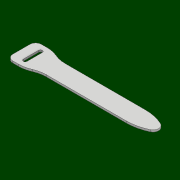
# Autodesk Inventor part: fastener_strap_t1
Saved by Autodesk Inventor 2018 (Build 220112000, 112)
## iProperties
Created: 2021-12-05
Part Number: fastener_strap_t1
Material: 一般
Document SubType Name: Modeling
Designer: gisen
Density: 1 g/cm^3
Appearance: 既定
Author: gisen
Autodesk Inventor part; units mm, degrees
ref_plane "YZ Plane" through (0, 0, 0) normal (1, 0, 0) x (0, 1, 0)
ref_plane "XZ Plane" through (0, 0, 0) normal (0, 1, 0) x (-1, 0, 0)
ref_plane "XY Plane" through (0, 0, 0) normal (0, 0, 1) x (1, 0, 0)
sketch "スケッチ1" plane through (0, 0, 0) normal (0, 0, 1) x (1, 0, 0)
  line L0 (0, 4) -> (0, -4) construction
  line L1 (-1, 4) -> (-1, -4)
  line L2 (1, -4) -> (1, 4)
  arc A0 (1, 4) -> (-1, 4) centre (0, 4) ccw
  arc A1 (-1, -4) -> (1, -4) centre (0, -4) ccw
  arc A2 (64.2706, 2.7176) -> (54, 5) centre (54, -19.25) ccw
  line L3 (54, 5) -> (12, 5)
  line L4 (-6, 7.5) -> (0, 7.5)
  arc A3 (6, 6.25) -> (0, 7.5) centre (0, -7.525) ccw
  arc A4 (6, 6.25) -> (12, 5) centre (12, 20.025) ccw
  line L5 (-6, 7.5) -> (-6, 0)
  line L6 (-6, 0) -> (66, 0) construction
  arc A5 (66, 0) -> (64.2706, 2.7176) centre (63, 0) ccw
  arc A6 (54, -5) -> (64.2706, -2.7176) centre (54, 19.25) ccw
  line L7 (54, -5) -> (12, -5)
  line L8 (-6, -7.5) -> (0, -7.5)
  arc A7 (12, -5) -> (6, -6.25) centre (12, -20.025) ccw
  line L9 (-6, -7.5) -> (-6, 0)
  arc A8 (64.2706, -2.7176) -> (66, 0) centre (63, 0) ccw
  arc A9 (0, -7.5) -> (6, -6.25) centre (0, 7.525) ccw
  point P0 (0, 0)
  point P1 (0, 0)
  point P2 (0, 5)
  point P3 (0, -5)
  dimension "d0" = 2
  dimension "d1" = 10
  dimension "d2" = 7.5
  dimension "d3" = 6
  dimension "d4" = 0
  dimension "d5" = 5
  dimension "d6" = 12
  dimension "d7" = 6
  dimension "d8" = 72
  dimension "d9" = 3
  dimension "d10" = 9
  constraints: 24 point on circle, 22 end point, 10 centre point, 9 symmetric about line, 9 tangent, 2 horizontal, 2 point on line, 2 vertical, 1 coincident, 1 midpoint, 1 parallel, 1 perpendicular, 4 other
  measures "d0" distance between parallel lines of L2 L1
  measures "d1" distance of point (0, -5) point (0, 5)
  measures "d2" distance between parallel lines of L6 L4
  measures "d3" distance between parallel lines of L0 L5
  measures "d4" distance from line of L0 L4.end
  measures "d5" distance from line of L3 point (0, 0)
  measures "d6" distance from line of L0 L3.end
  measures "d7" distance from line of L0 A3.start
  measures "d8" distance of L6.end L5.end
  measures "d9" distance of L6.end A5.centre
  measures "d10" horizontal distance of A5.centre L3.start
extrude "押し出し1" add sketch "スケッチ1" along normal blind 1
fillet "フィレット1" radius 3 2 edges at (-6, 7.5, 0.5) (-6, -7.5, 0.5)
